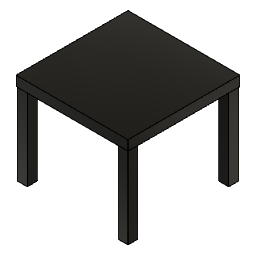
LackTableBrace_v3 (Autodesk Fusion 360 archive; units mm, degrees)
design "LackTable"
Autodesk Fusion 360 part; units mm, degrees
sketch "Sketch1" plane through (0, 0, 0) normal (0, 0, 1) x (1, 0, 0) in component "Top"
  line L0 (275, 275) -> (-275, 275)
  line L1 (-275, 275) -> (-275, -275)
  line L2 (-275, -275) -> (275, -275)
  line L3 (275, -275) -> (275, 275)
  line L4 (275, 275) -> (-275, -275) construction
  line L5 (-275, 275) -> (275, -275) construction
  dimension "d1" = 550
  dimension "d2" = 550
  constraint horizontal L0
  constraint perpendicular L0 L1
  constraint parallel L0 L2
  constraint parallel L1 L3
  constraint coincident L4 origin
  constraint coincident L5 origin
  measures "d1" distance of L1.end L2.end
  measures "d2" distance of L0.end L1.end
extrude "Extrude1" add sketch "Sketch1" along normal blind 50 makes body 1 in component "Top"
sketch "Sketch1 (2)" plane through (0, 0, 0) normal (0, 0, -1) x (1, 0, 0) in component "Leg"
  line L0 (275, -275) -> (275, 275)
  line L1 (275, 275) -> (-275, 275)
  line L2 (-275, 275) -> (-275, -275)
  line L3 (-275, -275) -> (275, -275)
  line L4 (323.0985, 293.2911) -> (373.0985, 293.2911)
  line L5 (373.0985, 293.2911) -> (373.0985, 243.2911)
  line L6 (373.0985, 243.2911) -> (323.0985, 243.2911)
  line L7 (323.0985, 243.2911) -> (323.0985, 293.2911)
  dimension "d5" = 50
  dimension "d6" = 50
  constraint horizontal L4
  constraint vertical L5
  constraint horizontal L6
  constraint vertical L7
  measures "d5" distance of L4.start L4.end
  measures "d6" distance of L4.start L6.end
extrude "Extrude1'" add sketch "Sketch1 (2)" along normal blind 400 separate body contours L4 L5 L6 L7 makes body 2 in component "Leg"
chamfer "Chamfer1" distance 1 angle 45 4 edges at (373.0985, -243.2911, -200) (323.0985, -243.2911, -200) (323.0985, -293.2911, -200) (373.0985, -293.2911, -200) on bodies 2 in component "Leg"
pattern_linear "持1" [suppressed] in component "Lega"
chamfer "Chamfer1'" distance 1.5 angle 45 4 edges at (0, 275, 0) (275, 0, 0) (0, -275, 0) (-275, 0, 0) on bodies 1 in component "Top"
chamfer "Chamfer2" distance 1 angle 45 4 edges at (-275, -275, 25.75) (-275, 275, 25.75) (275, 275, 25.75) (275, -275, 25.75) on bodies 1 in component "Top"
component "Top" placed x (1, 0, 0) y (0, 1, 0) z (0, 0, 1) at (0, 0, 0)
component "Lega" placed x (1, 0, 0) y (0, 1, 0) z (0, 0, 1) at (0, 0, 0)
component "Leg" placed x (1, 0, 0) y (0, 1, 0) z (0, 0, 1) at (-100.5985, 20.7911, 0) in component "Lega"
component "Leg" placed x (1, 0, 0) y (0, 1, 0) z (0, 0, 1) at (-595.5985, 20.7911, 0) in component "Lega"
component "Leg" placed x (1, 0, 0) y (0, 1, 0) z (0, 0, 1) at (-100.5985, 515.7911, 0) in component "Lega"
component "Leg" placed x (1, 0, 0) y (0, 1, 0) z (0, 0, 1) at (-595.5985, 515.7911, 0) in component "Lega"
